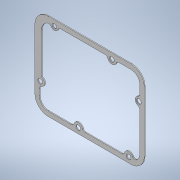
# Autodesk Inventor part: Прокладка
Saved by Autodesk Inventor 2021 (Build 250183000, 183)
## iProperties
Created: 2021-04-27
Part Number: Прокладка
Material: Типовые
Document SubType Name: Modeling
Designer: Данил
Density: 1 g/cm^3
Appearance: По умолчанию
Author: Данил
Autodesk Inventor part; units mm, degrees
ref_plane "YZ Plane" through (0, 0, 0) normal (1, 0, 0) x (0, 1, 0)
ref_plane "XZ Plane" through (0, 0, 0) normal (0, 1, 0) x (-1, 0, 0)
ref_plane "XY Plane" through (0, 0, 0) normal (0, 0, 1) x (1, 0, 0)
sketch "Эскиз1" plane through (0, 0, 0) normal (0, 0, 1) x (1, 0, 0)
  circle A0 centre (127, 6) radius 5.25
  circle A1 centre (104, -114) radius 5.15
  circle A2 centre (-10, -114) radius 5.25
  arc A3 (-108, -96) -> (-78, -126) centre (-78, -96) ccw
  line L0 (109, -126) -> (-78, -126)
  arc A4 (109, -126) -> (139, -96) centre (109, -96) ccw
  line L1 (139, 40) -> (139, -96)
  arc A5 (139, 40) -> (109, 70.2105) centre (109.0007, 40.2105) ccw
  line L2 (52, 70.2105) -> (109, 70.2105)
  line L3 (-77.5789, 70.2105) -> (52, 70.2105)
  arc A6 (-102, 58) -> (-108, 40) centre (-78, 40) ccw
  line L4 (-108, -96) -> (-108, 40)
  circle A7 centre (-64, 58) radius 5.15
  circle A8 centre (-96, -66) radius 5.25
  circle A9 centre (66, 58) radius 5.25
  line L5 (129.1156, -8.9658) -> (129.1156, -95.4445)
  arc A10 (122.1506, -110.6662) -> (129.1156, -95.4445) centre (109, -95.4445) ccw
  arc A11 (112.8925, -108.8704) -> (122.1506, -110.6662) centre (118.2281, -106.1259) ccw
  arc A12 (112.8925, -108.8704) -> (94.2992, -111.0168) centre (104, -113.4445) ccw
  arc A13 (88.4787, -115.5601) -> (94.2992, -111.0168) centre (88.4787, -109.5601) ccw
  line L6 (88.4787, -115.5601) -> (5.5213, -115.5601)
  arc A14 (-0.2992, -111.0168) -> (5.5213, -115.5601) centre (5.5213, -109.5601) ccw
  arc A15 (-0.2992, -111.0168) -> (-19.7008, -111.0168) centre (-10, -113.4445) ccw
  arc A16 (-25.5213, -115.5601) -> (-19.7008, -111.0168) centre (-25.5213, -109.5601) ccw
  line L7 (-25.5213, -115.5601) -> (-78, -115.5601)
  arc A17 (-98.1156, -95.4445) -> (-78, -115.5601) centre (-78, -95.4445) ccw
  line L8 (-98.1156, -95.4445) -> (-98.1156, -80.9658)
  arc A18 (-93.5722, -75.1454) -> (-98.1156, -80.9658) centre (-92.1156, -80.9658) ccw
  arc A19 (-93.5722, -75.1454) -> (-93, -55.9051) centre (-96, -65.4445) ccw
  line L9 (-93, -55.9051) -> (-93, 35.5555)
  arc A20 (56.5572, 55.6619) -> (53.2581, 59.6498) centre (50.7367, 54.2052) ccw
  arc A21 (56.5572, 55.6619) -> (75.9589, 55.6619) centre (66.2581, 58.0897) ccw
  arc A22 (81.7794, 59.6498) -> (75.9589, 55.6619) centre (81.6122, 53.6521) ccw
  line L10 (81.7794, 59.6498) -> (109.2581, 59.6498)
  arc A23 (129.3736, 39.5342) -> (109.2581, 59.6498) centre (109.2581, 39.5342) ccw
  line L11 (129.3736, 39.5342) -> (129.3736, 21.0555)
  arc A24 (124.8303, 15.235) -> (129.3736, 21.0555) centre (123.3736, 21.0555) ccw
  arc A25 (124.8303, 15.235) -> (124.5722, -3.1454) centre (128.6409, 5.9895) ccw
  arc A26 (129.1156, -8.9658) -> (124.5722, -3.1454) centre (123.1156, -8.9658) ccw
  line L12 (53.2581, 59.6498) -> (-48.8888, 59.6498)
  arc A27 (-48.8888, 59.6498) -> (-55.9983, 54.8231) centre (-48.8888, 52.0004) ccw
  arc A28 (-71.1639, 53.2252) -> (-55.9983, 54.8231) centre (-64, 58) ccw
  arc A29 (-71.1639, 53.2252) -> (-81.1576, 55.6548) centre (-77.4795, 49.0158) ccw
  arc A30 (-81.1576, 55.6548) -> (-93, 35.5555) centre (-70.0221, 35.5555) ccw
  arc A31 (-77.5789, 70.2105) -> (-102, 58) centre (-77.5789, 39.6842) ccw
  point P0 (0, 0)
  point P1 (0, 0)
  constraints: 52 point on circle, 32 centre point, 26 end point, 7 tangent, 1 coincident, 1 horizontal, 1 horizontal alignment
extrude "Выдавливание1" add sketch "Эскиз1" along normal mid plane 2
